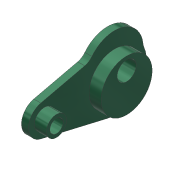
# Autodesk Inventor part: UPPER_LEG_BELT_TENSIONER
Saved by Autodesk Inventor 2019.4 (Build 234330000, 330)
## iProperties
Created: 2019-11-13
Part Number: UPPER_LEG_BELT_TENSIONER
Material: 一般
Document SubType Name: Modeling
Designer: y6tada
Density: 1 g/cm^3
Appearance: 滑らか - 濃い海緑
Mass: 0.229639 g
Surface Area: 5.47922 cm^2
Volume: 0.229639 cm^3
Author: y6tada
Autodesk Inventor part; units mm, degrees
ref_plane "YZ Plane" through (0, 0, 0) normal (1, 0, 0) x (0, 1, 0)
ref_plane "XZ Plane" through (0, 0, 0) normal (0, 1, 0) x (-1, 0, 0)
ref_plane "XY Plane" through (0, 0, 0) normal (0, 0, 1) x (1, 0, 0)
sketch "スケッチ1" plane through (0, 0, 0) normal (1, 0, 0) x (0, 1, 0)
  line L0 (0, 0) -> (0, -11) construction
  arc A0 (2.4346, 0.5682) -> (-2.4346, 0.5682) centre (0, 0) ccw
  circle A1 centre (0, -11) radius 4 construction
  line L1 (-2.4346, 0.5682) -> (-4.8692, -9.8636)
  arc A2 (0, -2.5) -> (2.4346, 0.5682) centre (0, 0) ccw construction
  arc A3 (-2.4346, 0.5682) -> (0, -2.5) centre (0, 0) ccw construction
  arc A4 (-4.8692, -9.8636) -> (1.9196, -15.6168) centre (0, -11) ccw
  arc A5 (-0.8211, -15.9321) -> (2.1875, -15.4961) centre (0, -11) ccw construction
  line L2 (2.4346, 0.5682) -> (4.043, -6.3238)
  arc A6 (2.476, -15.4748) -> (4.7628, -7.448) centre (2, -11) ccw
  line L3 (0, -11) -> (2, -11) construction
  arc A7 (0, -6) -> (-4.8692, -9.8636) centre (0, -11) ccw construction
  arc A8 (4.043, -6.3238) -> (4.7628, -7.448) centre (5.9907, -5.8693) ccw
  arc A9 (2.476, -15.4748) -> (1.9196, -15.6168) centre (2.6875, -17.4635) ccw
  point P0 (4.221, -7.0863)
  dimension "d1" = 11
  dimension "d2" = 8
  dimension "d4" = 2.5
  dimension "d39" = 5
  dimension "d54" = 2
  dimension "d55" = 4.5
  dimension "d56" = 2
  constraints: 22 point on circle, 11 tangent, 10 centre point, 8 end point, 2 coincident, 2 point on line, 1 concentric, 1 equal radius, 1 perpendicular, 1 vertical
  measures "d1" distance of L0.start L0.end
  measures "d2" diameter of A1
  measures "d4" radius of A0
  measures "d39" radius of A4
  measures "d54" distance of L3.start L3.end
  measures "d55" radius of A6
  measures "d56" radius of A8
extrude "押し出し1" add sketch "スケッチ1" along normal blind 1.1
sketch "スケッチ2" plane through (1.1, 0, 0) normal (1, 0, 0) x (0, 0, -1)
  circle A0 centre (0, 0) radius 1.575
  circle A1 centre (11, 0) radius 4
  line L0 (0, 0) -> (11, 0) construction
  arc A2 (9.8636, -4.8692) -> (15.6168, 1.9196) centre (11, 0) ccw construction
  point P0 (8.75, 4.8412)
  dimension "d12" = 3.15
  dimension "d13" = 8
  constraints: 2 centre point, 2 end point, 1 coincident, 1 horizontal, 2 other
  measures "d12" diameter of A0
  measures "d13" diameter of A1
extrude "押し出し2" add sketch "スケッチ2" along normal blind 1.9
sketch "スケッチ3" plane through (1.1, 0, 0) normal (1, 0, 0) x (0, 0, -1)
  point P0 (0, 0)
sketch "スケッチ4" plane through (0, 0, 0) normal (-1, 0, 0) x (0, 0, 1)
  arc A0 (0.5682, -2.4346) -> (0.5682, 2.4346) centre (0, 0) ccw construction
  arc A1 (-15.6168, 1.9196) -> (-9.8636, -4.8692) centre (-11, 0) ccw construction
  line L0 (-11, 0) -> (-11, 2) construction
  dimension "d53" = 2
  constraints: 2 coincident, 2 end point, 1 vertical
  measures "d53" distance of L0.start L0.end
hole "穴3" at (0, 0, 0) direction (1, 0, 0) diameter 2.1 end through all clearance for "Countersunk Flat Head Screw ISO 2009/7046" size "M2" standard "ISO"
hole "穴4" at (0, 2, -11) direction (1, 0, 0) diameter 2.99 end through all
